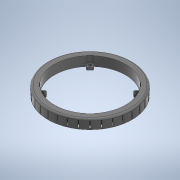
# Autodesk Inventor part: tsop_head_v2
Saved by Autodesk Inventor 2020 (Build 240168000, 168)
## iProperties
Created: 2024-03-11
Part Number: tsop_head_v2
Material: Типовые
Document SubType Name: Modeling
Designer: 4s
Density: 1 g/cm^3
Appearance: Гладкая — черная
Author: 4s
Autodesk Inventor part; units mm, degrees
ref_plane "YZ Plane" through (0, 0, 0) normal (1, 0, 0) x (0, 1, 0)
ref_plane "XZ Plane" through (0, 0, 0) normal (0, 1, 0) x (-1, 0, 0)
ref_plane "XY Plane" through (0, 0, 0) normal (0, 0, 1) x (1, 0, 0)
sketch "Эскиз1" plane through (0, 0, 0) normal (0, 1, 0) x (-1, 0, 0)
  circle A0 centre (0, 0) radius 44 construction
  line L0 (46.1, 2.85) -> (42.7, 2.85)
  line L1 (42.7, 2.85) -> (42.7, -2.85)
  line L2 (42.7, -2.85) -> (46.1, -2.85)
  line L3 (48.1, -0.85) -> (48.1, 0.85)
  line L4 (0, 0) -> (44, 0) construction
  line L5 (0, 0) -> (0, -44) construction
  circle A1 centre (0, 0) radius 49 construction
  circle A2 centre (0, 0) radius 42 construction
  circle A3 centre (0, 0) radius 39 construction
  arc A4 (48.1, 0.85) -> (46.1, 2.85) centre (46.1, 0.85) ccw
  arc A5 (46.1, -2.85) -> (48.1, -0.85) centre (46.1, -0.85) ccw
  line L6 (0, 0) -> (48.1, -0.4908) construction
  line L7 (0, 0) -> (48.1, 0.4908) construction
  line L8 (48.1, 0.4908) -> (48.9974, 0.5)
  line L9 (48.1, -0.4908) -> (48.9974, -0.5)
  line L10 (48.9974, 0.5) -> (49.2908, 0.1398)
  line L11 (49.2908, 0.1398) -> (48.9974, -0.5)
  arc A6 (48.9974, -0.5) -> (48.9974, 0.5) centre (0, 0) ccw
  point P0 (48.1, 2.85)
  point P1 (48.1, -2.85)
  point P2 (49, 0)
  dimension "d0" = 88
  dimension "d1" = 5.7
  dimension "d2" = 1.3
  dimension "d3" = 5.4
  dimension "d4" = 98
  dimension "d5" = 84
  dimension "d6" = 78
  dimension "d16" = 2
  dimension "d17" = 1
  constraints: 24 end point, 11 point on circle, 7 centre point, 6 point on line, 5 coincident, 4 tangent, 2 collinear, 2 horizontal, 2 parallel, 2 perpendicular, 1 equal radius, 1 symmetric about line, 1 other
  measures "d0" diameter of A0
  measures "d1" distance of point (48.1, -2.85) point (48.1, 2.85)
  measures "d2" distance from line of L4.end L1
  measures "d3" distance of L1.end point (48.1, -2.85)
  measures "d4" diameter of A1
  measures "d5" diameter of A2
  measures "d6" diameter of A3
  measures "d16" radius of A4
  measures "d17" distance of L8.end L9.end
sketch "Эскиз2" plane through (0, 0, 0) normal (0, 1, 0) x (-1, 0, 0)
  circle A0 centre (0, 0) radius 49
  circle A1 centre (0, 0) radius 42
  dimension "d7" = 98
  dimension "d8" = 84
  constraints: 2 centre point, 2 coincident
  measures "d7" diameter of A0
  measures "d8" diameter of A1
extrude "Выдавливание1" add sketch "Эскиз2" along normal blind 10
extrude "Выдавливание2" cut sketch "Эскиз1" along normal blind 10 contours A4 L3 A5 L2 L1 L0 | L10 L11 A6
pattern_circular "Круговой массив1" count 32 over 360 about axis through (0, 0, 0) along (0, 1, 0) of "Выдавливание2"
sketch "Эскиз3" plane through (0, 10, 0) normal (0, 1, 0) x (1, 0, 0)
  line L0 (-48.1, -0.85) -> (-48.1, 0.85) construction
  arc A0 (-46.1, 2.85) -> (-48.1, 0.85) centre (-46.1, 0.85) ccw construction
  line L1 (-46.1, 2.85) -> (-42.7, 2.85) construction
  line L2 (-42.7, 2.85) -> (-42.7, -2.85) construction
  line L3 (-42.7, -2.85) -> (-46.1, -2.85) construction
  arc A1 (-48.1, -0.85) -> (-46.1, -2.85) centre (-46.1, -0.85) ccw construction
  line L4 (-47.0099, -10.2175) -> (-47.3416, -8.5502) construction
  arc A2 (-45.7702, -6.1984) -> (-47.3416, -8.5502) centre (-45.38, -8.16) ccw construction
  line L5 (-45.7702, -6.1984) -> (-42.4355, -5.5351) construction
  line L6 (-42.4355, -5.5351) -> (-41.3235, -11.1256) construction
  line L7 (-41.3235, -11.1256) -> (-44.6582, -11.7889) construction
  arc A3 (-47.0099, -10.2175) -> (-44.6582, -11.7889) centre (-45.0484, -9.8273) ccw construction
  line L8 (-44.1133, -19.1924) -> (-44.7639, -17.6218) construction
  arc A4 (-43.6815, -15.0086) -> (-44.7639, -17.6218) centre (-42.9161, -16.8564) ccw construction
  line L9 (-43.6815, -15.0086) -> (-40.5403, -13.7075) construction
  line L10 (-40.5403, -13.7075) -> (-38.359, -18.9736) construction
  line L11 (-38.359, -18.9736) -> (-41.5002, -20.2748) construction
  arc A5 (-44.1133, -19.1924) -> (-41.5002, -20.2748) centre (-42.2656, -18.427) ccw construction
  line L12 (-39.5215, -27.4297) -> (-40.4659, -26.0162) construction
  arc A6 (-39.9141, -23.2421) -> (-40.4659, -26.0162) centre (-38.803, -24.905) ccw construction
  line L13 (-39.9141, -23.2421) -> (-37.0871, -21.3532) construction
  line L14 (-37.0871, -21.3532) -> (-33.9204, -26.0925) construction
  line L15 (-33.9204, -26.0925) -> (-36.7474, -27.9815) construction
  arc A7 (-39.5215, -27.4297) -> (-36.7474, -27.9815) centre (-37.8585, -26.3185) ccw construction
  line L16 (-33.4108, -34.6129) -> (-34.6129, -33.4108) construction
  arc A8 (-34.6129, -30.5824) -> (-34.6129, -33.4108) centre (-33.1987, -31.9966) ccw construction
  line L17 (-34.6129, -30.5824) -> (-32.2087, -28.1782) construction
  line L18 (-32.2087, -28.1782) -> (-28.1782, -32.2087) construction
  line L19 (-28.1782, -32.2087) -> (-30.5824, -34.6129) construction
  arc A9 (-33.4108, -34.6129) -> (-30.5824, -34.6129) centre (-31.9966, -33.1987) ccw construction
  line L20 (-26.0162, -40.4659) -> (-27.4297, -39.5215) construction
  arc A10 (-27.9815, -36.7474) -> (-27.4297, -39.5215) centre (-26.3185, -37.8585) ccw construction
  line L21 (-27.9815, -36.7474) -> (-26.0925, -33.9204) construction
  line L22 (-26.0925, -33.9204) -> (-21.3532, -37.0871) construction
  line L23 (-21.3532, -37.0871) -> (-23.2421, -39.9141) construction
  arc A11 (-26.0162, -40.4659) -> (-23.2421, -39.9141) centre (-24.905, -38.803) ccw construction
  line L24 (-17.6218, -44.7639) -> (-19.1924, -44.1133) construction
  arc A12 (-20.2748, -41.5002) -> (-19.1924, -44.1133) centre (-18.427, -42.2656) ccw construction
  line L25 (-20.2748, -41.5002) -> (-18.9736, -38.359) construction
  line L26 (-18.9736, -38.359) -> (-13.7075, -40.5403) construction
  line L27 (-13.7075, -40.5403) -> (-15.0086, -43.6815) construction
  arc A13 (-17.6218, -44.7639) -> (-15.0086, -43.6815) centre (-16.8564, -42.9161) ccw construction
  line L28 (-8.5502, -47.3416) -> (-10.2175, -47.0099) construction
  arc A14 (-11.7889, -44.6582) -> (-10.2175, -47.0099) centre (-9.8273, -45.0484) ccw construction
  line L29 (-11.7889, -44.6582) -> (-11.1256, -41.3235) construction
  line L30 (-11.1256, -41.3235) -> (-5.5351, -42.4355) construction
  line L31 (-5.5351, -42.4355) -> (-6.1984, -45.7702) construction
  arc A15 (-8.5502, -47.3416) -> (-6.1984, -45.7702) centre (-8.16, -45.38) ccw construction
  line L32 (0.85, -48.1) -> (-0.85, -48.1) construction
  arc A16 (-2.85, -46.1) -> (-0.85, -48.1) centre (-0.85, -46.1) ccw construction
  line L33 (-2.85, -46.1) -> (-2.85, -42.7) construction
  line L34 (-2.85, -42.7) -> (2.85, -42.7) construction
  line L35 (2.85, -42.7) -> (2.85, -46.1) construction
  arc A17 (0.85, -48.1) -> (2.85, -46.1) centre (0.85, -46.1) ccw construction
  line L36 (10.2175, -47.0099) -> (8.5502, -47.3416) construction
  arc A18 (6.1984, -45.7702) -> (8.5502, -47.3416) centre (8.16, -45.38) ccw construction
  line L37 (6.1984, -45.7702) -> (5.5351, -42.4355) construction
  line L38 (5.5351, -42.4355) -> (11.1256, -41.3235) construction
  line L39 (11.1256, -41.3235) -> (11.7889, -44.6582) construction
  arc A19 (10.2175, -47.0099) -> (11.7889, -44.6582) centre (9.8273, -45.0484) ccw construction
  line L40 (19.1924, -44.1133) -> (17.6218, -44.7639) construction
  arc A20 (15.0086, -43.6815) -> (17.6218, -44.7639) centre (16.8564, -42.9161) ccw construction
  line L41 (15.0086, -43.6815) -> (13.7075, -40.5403) construction
  line L42 (13.7075, -40.5403) -> (18.9736, -38.359) construction
  line L43 (18.9736, -38.359) -> (20.2748, -41.5002) construction
  arc A21 (19.1924, -44.1133) -> (20.2748, -41.5002) centre (18.427, -42.2656) ccw construction
  line L44 (27.4297, -39.5215) -> (26.0162, -40.4659) construction
  arc A22 (23.2421, -39.9141) -> (26.0162, -40.4659) centre (24.905, -38.803) ccw construction
  line L45 (23.2421, -39.9141) -> (21.3532, -37.0871) construction
  line L46 (21.3532, -37.0871) -> (26.0925, -33.9204) construction
  line L47 (26.0925, -33.9204) -> (27.9815, -36.7474) construction
  arc A23 (27.4297, -39.5215) -> (27.9815, -36.7474) centre (26.3185, -37.8585) ccw construction
  line L48 (34.6129, -33.4108) -> (33.4108, -34.6129) construction
  arc A24 (30.5824, -34.6129) -> (33.4108, -34.6129) centre (31.9966, -33.1987) ccw construction
  line L49 (30.5824, -34.6129) -> (28.1782, -32.2087) construction
  line L50 (28.1782, -32.2087) -> (32.2087, -28.1782) construction
  line L51 (32.2087, -28.1782) -> (34.6129, -30.5824) construction
  arc A25 (34.6129, -33.4108) -> (34.6129, -30.5824) centre (33.1987, -31.9966) ccw construction
  line L52 (40.4659, -26.0162) -> (39.5215, -27.4297) construction
  arc A26 (36.7474, -27.9815) -> (39.5215, -27.4297) centre (37.8585, -26.3185) ccw construction
  line L53 (36.7474, -27.9815) -> (33.9204, -26.0925) construction
  line L54 (33.9204, -26.0925) -> (37.0871, -21.3532) construction
  line L55 (37.0871, -21.3532) -> (39.9141, -23.2421) construction
  arc A27 (40.4659, -26.0162) -> (39.9141, -23.2421) centre (38.803, -24.905) ccw construction
  line L56 (44.7639, -17.6218) -> (44.1133, -19.1924) construction
  arc A28 (41.5002, -20.2748) -> (44.1133, -19.1924) centre (42.2656, -18.427) ccw construction
  line L57 (41.5002, -20.2748) -> (38.359, -18.9736) construction
  line L58 (38.359, -18.9736) -> (40.5403, -13.7075) construction
  line L59 (40.5403, -13.7075) -> (43.6815, -15.0086) construction
  arc A29 (44.7639, -17.6218) -> (43.6815, -15.0086) centre (42.9161, -16.8564) ccw construction
  line L60 (47.3416, -8.5502) -> (47.0099, -10.2175) construction
  arc A30 (44.6582, -11.7889) -> (47.0099, -10.2175) centre (45.0484, -9.8273) ccw construction
  line L61 (44.6582, -11.7889) -> (41.3235, -11.1256) construction
  line L62 (41.3235, -11.1256) -> (42.4355, -5.5351) construction
  line L63 (42.4355, -5.5351) -> (45.7702, -6.1984) construction
  arc A31 (47.3416, -8.5502) -> (45.7702, -6.1984) centre (45.38, -8.16) ccw construction
  line L64 (48.1, 0.85) -> (48.1, -0.85) construction
  arc A32 (46.1, -2.85) -> (48.1, -0.85) centre (46.1, -0.85) ccw construction
  line L65 (46.1, -2.85) -> (42.7, -2.85) construction
  line L66 (42.7, -2.85) -> (42.7, 2.85) construction
  line L67 (42.7, 2.85) -> (46.1, 2.85) construction
  arc A33 (48.1, 0.85) -> (46.1, 2.85) centre (46.1, 0.85) ccw construction
  line L68 (47.0099, 10.2175) -> (47.3416, 8.5502) construction
  arc A34 (45.7702, 6.1984) -> (47.3416, 8.5502) centre (45.38, 8.16) ccw construction
  line L69 (45.7702, 6.1984) -> (42.4355, 5.5351) construction
  line L70 (42.4355, 5.5351) -> (41.3235, 11.1256) construction
  line L71 (41.3235, 11.1256) -> (44.6582, 11.7889) construction
  arc A35 (47.0099, 10.2175) -> (44.6582, 11.7889) centre (45.0484, 9.8273) ccw construction
  line L72 (44.1133, 19.1924) -> (44.7639, 17.6218) construction
  arc A36 (43.6815, 15.0086) -> (44.7639, 17.6218) centre (42.9161, 16.8564) ccw construction
  line L73 (43.6815, 15.0086) -> (40.5403, 13.7075) construction
  line L74 (40.5403, 13.7075) -> (38.359, 18.9736) construction
  line L75 (38.359, 18.9736) -> (41.5002, 20.2748) construction
  arc A37 (44.1133, 19.1924) -> (41.5002, 20.2748) centre (42.2656, 18.427) ccw construction
  line L76 (39.5215, 27.4297) -> (40.4659, 26.0162) construction
  arc A38 (39.9141, 23.2421) -> (40.4659, 26.0162) centre (38.803, 24.905) ccw construction
  line L77 (39.9141, 23.2421) -> (37.0871, 21.3532) construction
  line L78 (37.0871, 21.3532) -> (33.9204, 26.0925) construction
  line L79 (33.9204, 26.0925) -> (36.7474, 27.9815) construction
  arc A39 (39.5215, 27.4297) -> (36.7474, 27.9815) centre (37.8585, 26.3185) ccw construction
  line L80 (33.4108, 34.6129) -> (34.6129, 33.4108) construction
  arc A40 (34.6129, 30.5824) -> (34.6129, 33.4108) centre (33.1987, 31.9966) ccw construction
  line L81 (34.6129, 30.5824) -> (32.2087, 28.1782) construction
  line L82 (32.2087, 28.1782) -> (28.1782, 32.2087) construction
  line L83 (28.1782, 32.2087) -> (30.5824, 34.6129) construction
  arc A41 (33.4108, 34.6129) -> (30.5824, 34.6129) centre (31.9966, 33.1987) ccw construction
  line L84 (26.0162, 40.4659) -> (27.4297, 39.5215) construction
  arc A42 (27.9815, 36.7474) -> (27.4297, 39.5215) centre (26.3185, 37.8585) ccw construction
  line L85 (27.9815, 36.7474) -> (26.0925, 33.9204) construction
  line L86 (26.0925, 33.9204) -> (21.3532, 37.0871) construction
  line L87 (21.3532, 37.0871) -> (23.2421, 39.9141) construction
  arc A43 (26.0162, 40.4659) -> (23.2421, 39.9141) centre (24.905, 38.803) ccw construction
  line L88 (17.6218, 44.7639) -> (19.1924, 44.1133) construction
  arc A44 (20.2748, 41.5002) -> (19.1924, 44.1133) centre (18.427, 42.2656) ccw construction
  line L89 (20.2748, 41.5002) -> (18.9736, 38.359) construction
  line L90 (18.9736, 38.359) -> (13.7075, 40.5403) construction
  line L91 (13.7075, 40.5403) -> (15.0086, 43.6815) construction
  arc A45 (17.6218, 44.7639) -> (15.0086, 43.6815) centre (16.8564, 42.9161) ccw construction
  line L92 (8.5502, 47.3416) -> (10.2175, 47.0099) construction
  arc A46 (11.7889, 44.6582) -> (10.2175, 47.0099) centre (9.8273, 45.0484) ccw construction
  line L93 (11.7889, 44.6582) -> (11.1256, 41.3235) construction
  line L94 (11.1256, 41.3235) -> (5.5351, 42.4355) construction
  line L95 (5.5351, 42.4355) -> (6.1984, 45.7702) construction
  arc A47 (8.5502, 47.3416) -> (6.1984, 45.7702) centre (8.16, 45.38) ccw construction
  line L96 (-0.85, 48.1) -> (0.85, 48.1) construction
  arc A48 (2.85, 46.1) -> (0.85, 48.1) centre (0.85, 46.1) ccw construction
  line L97 (2.85, 46.1) -> (2.85, 42.7) construction
  line L98 (2.85, 42.7) -> (-2.85, 42.7) construction
  line L99 (-2.85, 42.7) -> (-2.85, 46.1) construction
  arc A49 (-0.85, 48.1) -> (-2.85, 46.1) centre (-0.85, 46.1) ccw construction
  line L100 (-10.2175, 47.0099) -> (-8.5502, 47.3416) construction
  arc A50 (-6.1984, 45.7702) -> (-8.5502, 47.3416) centre (-8.16, 45.38) ccw construction
  line L101 (-6.1984, 45.7702) -> (-5.5351, 42.4355) construction
  line L102 (-5.5351, 42.4355) -> (-11.1256, 41.3235) construction
  line L103 (-11.1256, 41.3235) -> (-11.7889, 44.6582) construction
  arc A51 (-10.2175, 47.0099) -> (-11.7889, 44.6582) centre (-9.8273, 45.0484) ccw construction
  line L104 (-19.1924, 44.1133) -> (-17.6218, 44.7639) construction
  arc A52 (-15.0086, 43.6815) -> (-17.6218, 44.7639) centre (-16.8564, 42.9161) ccw construction
  line L105 (-15.0086, 43.6815) -> (-13.7075, 40.5403) construction
  line L106 (-13.7075, 40.5403) -> (-18.9736, 38.359) construction
  line L107 (-18.9736, 38.359) -> (-20.2748, 41.5002) construction
  arc A53 (-19.1924, 44.1133) -> (-20.2748, 41.5002) centre (-18.427, 42.2656) ccw construction
  line L108 (-27.4297, 39.5215) -> (-26.0162, 40.4659) construction
  arc A54 (-23.2421, 39.9141) -> (-26.0162, 40.4659) centre (-24.905, 38.803) ccw construction
  line L109 (-23.2421, 39.9141) -> (-21.3532, 37.0871) construction
  line L110 (-21.3532, 37.0871) -> (-26.0925, 33.9204) construction
  line L111 (-26.0925, 33.9204) -> (-27.9815, 36.7474) construction
  arc A55 (-27.4297, 39.5215) -> (-27.9815, 36.7474) centre (-26.3185, 37.8585) ccw construction
  line L112 (-34.6129, 33.4108) -> (-33.4108, 34.6129) construction
  arc A56 (-30.5824, 34.6129) -> (-33.4108, 34.6129) centre (-31.9966, 33.1987) ccw construction
  line L113 (-30.5824, 34.6129) -> (-28.1782, 32.2087) construction
  line L114 (-28.1782, 32.2087) -> (-32.2087, 28.1782) construction
  line L115 (-32.2087, 28.1782) -> (-34.6129, 30.5824) construction
  arc A57 (-34.6129, 33.4108) -> (-34.6129, 30.5824) centre (-33.1987, 31.9966) ccw construction
  line L116 (-40.4659, 26.0162) -> (-39.5215, 27.4297) construction
  arc A58 (-36.7474, 27.9815) -> (-39.5215, 27.4297) centre (-37.8585, 26.3185) ccw construction
  line L117 (-36.7474, 27.9815) -> (-33.9204, 26.0925) construction
  line L118 (-33.9204, 26.0925) -> (-37.0871, 21.3532) construction
  line L119 (-37.0871, 21.3532) -> (-39.9141, 23.2421) construction
  arc A59 (-40.4659, 26.0162) -> (-39.9141, 23.2421) centre (-38.803, 24.905) ccw construction
  line L120 (-44.7639, 17.6218) -> (-44.1133, 19.1924) construction
  arc A60 (-41.5002, 20.2748) -> (-44.1133, 19.1924) centre (-42.2656, 18.427) ccw construction
  line L121 (-41.5002, 20.2748) -> (-38.359, 18.9736) construction
  line L122 (-38.359, 18.9736) -> (-40.5403, 13.7075) construction
  line L123 (-40.5403, 13.7075) -> (-43.6815, 15.0086) construction
  arc A61 (-44.7639, 17.6218) -> (-43.6815, 15.0086) centre (-42.9161, 16.8564) ccw construction
  line L124 (-47.3416, 8.5502) -> (-47.0099, 10.2175) construction
  arc A62 (-44.6582, 11.7889) -> (-47.0099, 10.2175) centre (-45.0484, 9.8273) ccw construction
  line L125 (-44.6582, 11.7889) -> (-41.3235, 11.1256) construction
  line L126 (-41.3235, 11.1256) -> (-42.4355, 5.5351) construction
  line L127 (-42.4355, 5.5351) -> (-45.7702, 6.1984) construction
  arc A63 (-47.3416, 8.5502) -> (-45.7702, 6.1984) centre (-45.38, 8.16) ccw construction
  circle A64 centre (0, 0) radius 42 projected
  circle A65 centre (0, 0) radius 49
  constraints: 1 centre point, 1 coincident
extrude "Выдавливание3" add sketch "Эскиз3" along normal blind 1
fillet "Сопряжение1" radius 2 1 edges at (-49, 11, 0)
extrude "Выдавливание4" cut sketch "Эскиз1" along normal blind 9 contours L8 A6 L9 L3
pattern_circular "Круговой массив2" count 32 over 360 about axis through (0, 0, 0) along (0, 1, 0) of "Выдавливание4"
fillet "Сопряжение2" radius 0.5 1 edges at (-47.1758, 9, -9.3838)
sketch "Эскиз4" plane through (0, 0, 0) normal (0, -1, 0) x (1, 0, 0)
  circle A0 centre (0, 0) radius 39 construction
  line L0 (0, 0) -> (-27.5772, -27.5772) construction
  line L1 (0, 0) -> (39, 0) construction
  circle A1 centre (-27.5772, -27.5772) radius 1.7
  line L2 (0, 0) -> (0, -39) construction
  circle A2 centre (27.5772, -27.5772) radius 1.7
  circle A3 centre (-27.5772, 27.5772) radius 1.7
  circle A4 centre (27.5772, 27.5772) radius 1.7
  line L3 (-31.9075, -27.3113) -> (-28.8146, -24.2184)
  line L4 (-27.3113, -31.9075) -> (-24.2184, -28.8146)
  circle A5 centre (0, 0) radius 42 construction
  circle A6 centre (0, 0) radius 47 construction
  circle A7 centre (0, 0) radius 42 construction
  line L5 (-26.6933, -24.2184) -> (-24.2184, -26.6933)
  arc A8 (-24.2184, -28.8146) -> (-24.2184, -26.6933) centre (-25.2791, -27.7539) ccw
  arc A9 (-26.6933, -24.2184) -> (-28.8146, -24.2184) centre (-27.7539, -25.2791) ccw
  arc A10 (-31.9075, -27.3113) -> (-27.3113, -31.9075) centre (0, 0) ccw
  point P0 (-39, 0)
  point P1 (0, 39)
  point P2 (-27.7539, -23.1577)
  point P3 (-23.1577, -27.7539)
  dimension "d27" = 78
  dimension "d28" = 135
  dimension "d29" = 3.4
  dimension "d30" = 6.5
  dimension "d31" = 3
  dimension "d32" = 1.5
  dimension "d33" = 42
  constraints: 12 end point, 11 point on circle, 8 centre point, 5 symmetric about line, 4 point on line, 4 tangent, 2 coincident, 1 equal length, 1 equal radius, 1 horizontal, 1 parallel, 1 vertical, 5 other
  measures "d27" diameter of A0
  measures "d28" angle of L0 L1
  measures "d29" diameter of A1
  measures "d30" distance between parallel lines of L3 L4
  measures "d31" distance from line of L0.end L5
  measures "d32" radius of A8
  measures "d33" radius of A10
extrude "Выдавливание5" add sketch "Эскиз4" along normal blind 0 and the other way blind 2.8 contours L3 A9 L5 A8 L4 A10
pattern_circular "Круговой массив3" count 4 over 360 about axis through (0, 0, 0) along (0, 1, 0) of "Выдавливание5"
sketch "Эскиз5" plane through (0, 0, 0) normal (0, -1, 0) x (1, 0, 0)
  circle A0 centre (0, 0) radius 47 construction
  line L0 (-47.08, -9.8653) -> (-47.9584, -10.0493) construction
  arc A1 (-47.9584, -10.0493) -> (-45.4591, -18.2886) centre (0, 0) ccw construction
  line L1 (-45.4591, -18.2886) -> (-44.6264, -17.9536) construction
  line L2 (-44.6264, -17.9536) -> (-44.7639, -17.6218) construction
  arc A2 (-43.6815, -15.0086) -> (-44.7639, -17.6218) centre (-42.9161, -16.8564) ccw construction
  line L3 (-43.6815, -15.0086) -> (-40.5403, -13.7075) construction
  line L4 (-40.5403, -13.7075) -> (-38.359, -18.9736) construction
  line L5 (-38.359, -18.9736) -> (-41.5002, -20.2748) construction
  arc A3 (-44.1133, -19.1924) -> (-41.5002, -20.2748) centre (-42.2656, -18.427) ccw construction
  line L6 (-44.1133, -19.1924) -> (-44.2508, -18.8606) construction
  line L7 (-44.2508, -18.8606) -> (-45.0764, -19.2125) construction
  arc A4 (-45.0764, -19.2125) -> (-41.0177, -26.8058) centre (0, 0) ccw construction
  line L8 (-41.0177, -26.8058) -> (-40.2664, -26.3148) construction
  line L9 (-40.2664, -26.3148) -> (-40.4659, -26.0162) construction
  arc A5 (-39.9141, -23.2421) -> (-40.4659, -26.0162) centre (-38.803, -24.905) ccw construction
  line L10 (-39.9141, -23.2421) -> (-37.0871, -21.3532) construction
  line L11 (-37.0871, -21.3532) -> (-33.9204, -26.0925) construction
  line L12 (-33.9204, -26.0925) -> (-36.7474, -27.9815) construction
  arc A6 (-39.5215, -27.4297) -> (-36.7474, -27.9815) centre (-37.8585, -26.3185) ccw construction
  line L13 (-39.5215, -27.4297) -> (-39.721, -27.131) construction
  line L14 (-39.721, -27.131) -> (-40.4621, -27.6373) construction
  arc A7 (-40.4621, -27.6373) -> (-35, -34.2929) centre (0, 0) ccw construction
  line L15 (-35, -34.2929) -> (-34.3589, -33.6648) construction
  line L16 (-34.3589, -33.6648) -> (-34.6129, -33.4108) construction
  arc A8 (-34.6129, -30.5824) -> (-34.6129, -33.4108) centre (-33.1987, -31.9966) ccw construction
  line L17 (-34.6129, -30.5824) -> (-32.2087, -28.1782) construction
  line L18 (-32.2087, -28.1782) -> (-28.1782, -32.2087) construction
  line L19 (-28.1782, -32.2087) -> (-30.5824, -34.6129) construction
  arc A9 (-33.4108, -34.6129) -> (-30.5824, -34.6129) centre (-31.9966, -33.1987) ccw construction
  line L20 (-33.4108, -34.6129) -> (-33.6648, -34.3589) construction
  line L21 (-33.6648, -34.3589) -> (-34.2929, -35) construction
  arc A10 (-34.2929, -35) -> (-27.6373, -40.4621) centre (0, 0) ccw construction
  line L22 (-27.6373, -40.4621) -> (-27.131, -39.721) construction
  line L23 (-27.131, -39.721) -> (-27.4297, -39.5215) construction
  arc A11 (-27.9815, -36.7474) -> (-27.4297, -39.5215) centre (-26.3185, -37.8585) ccw construction
  line L24 (-27.9815, -36.7474) -> (-26.0925, -33.9204) construction
  line L25 (-26.0925, -33.9204) -> (-21.3532, -37.0871) construction
  line L26 (-21.3532, -37.0871) -> (-23.2421, -39.9141) construction
  arc A12 (-26.0162, -40.4659) -> (-23.2421, -39.9141) centre (-24.905, -38.803) ccw construction
  line L27 (-26.0162, -40.4659) -> (-26.3148, -40.2664) construction
  line L28 (-26.3148, -40.2664) -> (-26.8058, -41.0177) construction
  arc A13 (-26.8058, -41.0177) -> (-19.2125, -45.0764) centre (0, 0) ccw construction
  line L29 (-19.2125, -45.0764) -> (-18.8606, -44.2508) construction
  line L30 (-18.8606, -44.2508) -> (-19.1924, -44.1133) construction
  arc A14 (-20.2748, -41.5002) -> (-19.1924, -44.1133) centre (-18.427, -42.2656) ccw construction
  line L31 (-20.2748, -41.5002) -> (-18.9736, -38.359) construction
  line L32 (-18.9736, -38.359) -> (-13.7075, -40.5403) construction
  line L33 (-13.7075, -40.5403) -> (-15.0086, -43.6815) construction
  arc A15 (-17.6218, -44.7639) -> (-15.0086, -43.6815) centre (-16.8564, -42.9161) ccw construction
  line L34 (-17.6218, -44.7639) -> (-17.9536, -44.6264) construction
  line L35 (-17.9536, -44.6264) -> (-18.2886, -45.4591) construction
  arc A16 (-18.2886, -45.4591) -> (-10.0493, -47.9584) centre (0, 0) ccw construction
  line L36 (-10.0493, -47.9584) -> (-9.8653, -47.08) construction
  line L37 (-9.8653, -47.08) -> (-10.2175, -47.0099) construction
  arc A17 (-11.7889, -44.6582) -> (-10.2175, -47.0099) centre (-9.8273, -45.0484) ccw construction
  line L38 (-11.7889, -44.6582) -> (-11.1256, -41.3235) construction
  line L39 (-11.1256, -41.3235) -> (-5.5351, -42.4355) construction
  line L40 (-5.5351, -42.4355) -> (-6.1984, -45.7702) construction
  arc A18 (-8.5502, -47.3416) -> (-6.1984, -45.7702) centre (-8.16, -45.38) ccw construction
  line L41 (-8.5502, -47.3416) -> (-8.9024, -47.2715) construction
  line L42 (-8.9024, -47.2715) -> (-9.0685, -48.1535) construction
  arc A19 (-9.0685, -48.1535) -> (-0.5, -48.9974) centre (0, 0) ccw construction
  line L43 (-0.5, -48.9974) -> (-0.4908, -48.1) construction
  line L44 (-0.4908, -48.1) -> (-0.85, -48.1) construction
  arc A20 (-2.85, -46.1) -> (-0.85, -48.1) centre (-0.85, -46.1) ccw construction
  line L45 (-2.85, -46.1) -> (-2.85, -42.7) construction
  line L46 (-2.85, -42.7) -> (2.85, -42.7) construction
  line L47 (2.85, -42.7) -> (2.85, -46.1) construction
  arc A21 (0.85, -48.1) -> (2.85, -46.1) centre (0.85, -46.1) ccw construction
  line L48 (0.85, -48.1) -> (0.4908, -48.1) construction
  line L49 (0.4908, -48.1) -> (0.5, -48.9974) construction
  arc A22 (0.5, -48.9974) -> (9.0685, -48.1535) centre (0, 0) ccw construction
  line L50 (9.0685, -48.1535) -> (8.9024, -47.2715) construction
  line L51 (8.9024, -47.2715) -> (8.5502, -47.3416) construction
  arc A23 (6.1984, -45.7702) -> (8.5502, -47.3416) centre (8.16, -45.38) ccw construction
  line L52 (6.1984, -45.7702) -> (5.5351, -42.4355) construction
  line L53 (5.5351, -42.4355) -> (11.1256, -41.3235) construction
  line L54 (11.1256, -41.3235) -> (11.7889, -44.6582) construction
  arc A24 (10.2175, -47.0099) -> (11.7889, -44.6582) centre (9.8273, -45.0484) ccw construction
  line L55 (10.2175, -47.0099) -> (9.8653, -47.08) construction
  line L56 (9.8653, -47.08) -> (10.0493, -47.9584) construction
  arc A25 (10.0493, -47.9584) -> (18.2886, -45.4591) centre (0, 0) ccw construction
  line L57 (18.2886, -45.4591) -> (17.9536, -44.6264) construction
  line L58 (17.9536, -44.6264) -> (17.6218, -44.7639) construction
  arc A26 (15.0086, -43.6815) -> (17.6218, -44.7639) centre (16.8564, -42.9161) ccw construction
  line L59 (15.0086, -43.6815) -> (13.7075, -40.5403) construction
  line L60 (13.7075, -40.5403) -> (18.9736, -38.359) construction
  line L61 (18.9736, -38.359) -> (20.2748, -41.5002) construction
  arc A27 (19.1924, -44.1133) -> (20.2748, -41.5002) centre (18.427, -42.2656) ccw construction
  line L62 (19.1924, -44.1133) -> (18.8606, -44.2508) construction
  line L63 (18.8606, -44.2508) -> (19.2125, -45.0764) construction
  arc A28 (19.2125, -45.0764) -> (26.8058, -41.0177) centre (0, 0) ccw construction
  line L64 (26.8058, -41.0177) -> (26.3148, -40.2664) construction
  line L65 (26.3148, -40.2664) -> (26.0162, -40.4659) construction
  arc A29 (23.2421, -39.9141) -> (26.0162, -40.4659) centre (24.905, -38.803) ccw construction
  line L66 (23.2421, -39.9141) -> (21.3532, -37.0871) construction
  line L67 (21.3532, -37.0871) -> (26.0925, -33.9204) construction
  line L68 (26.0925, -33.9204) -> (27.9815, -36.7474) construction
  arc A30 (27.4297, -39.5215) -> (27.9815, -36.7474) centre (26.3185, -37.8585) ccw construction
  line L69 (27.4297, -39.5215) -> (27.131, -39.721) construction
  line L70 (27.131, -39.721) -> (27.6373, -40.4621) construction
  arc A31 (27.6373, -40.4621) -> (34.2929, -35) centre (0, 0) ccw construction
  line L71 (34.2929, -35) -> (33.6648, -34.3589) construction
  line L72 (33.6648, -34.3589) -> (33.4108, -34.6129) construction
  arc A32 (30.5824, -34.6129) -> (33.4108, -34.6129) centre (31.9966, -33.1987) ccw construction
  line L73 (30.5824, -34.6129) -> (28.1782, -32.2087) construction
  line L74 (28.1782, -32.2087) -> (32.2087, -28.1782) construction
  line L75 (32.2087, -28.1782) -> (34.6129, -30.5824) construction
  arc A33 (34.6129, -33.4108) -> (34.6129, -30.5824) centre (33.1987, -31.9966) ccw construction
  line L76 (34.6129, -33.4108) -> (34.3589, -33.6648) construction
  line L77 (34.3589, -33.6648) -> (35, -34.2929) construction
  arc A34 (35, -34.2929) -> (40.4621, -27.6373) centre (0, 0) ccw construction
  line L78 (40.4621, -27.6373) -> (39.721, -27.131) construction
  line L79 (39.721, -27.131) -> (39.5215, -27.4297) construction
  arc A35 (36.7474, -27.9815) -> (39.5215, -27.4297) centre (37.8585, -26.3185) ccw construction
  line L80 (36.7474, -27.9815) -> (33.9204, -26.0925) construction
  line L81 (33.9204, -26.0925) -> (37.0871, -21.3532) construction
  line L82 (37.0871, -21.3532) -> (39.9141, -23.2421) construction
  arc A36 (40.4659, -26.0162) -> (39.9141, -23.2421) centre (38.803, -24.905) ccw construction
  line L83 (40.4659, -26.0162) -> (40.2664, -26.3148) construction
  line L84 (40.2664, -26.3148) -> (41.0177, -26.8058) construction
  arc A37 (41.0177, -26.8058) -> (45.0764, -19.2125) centre (0, 0) ccw construction
  line L85 (45.0764, -19.2125) -> (44.2508, -18.8606) construction
  line L86 (44.2508, -18.8606) -> (44.1133, -19.1924) construction
  arc A38 (41.5002, -20.2748) -> (44.1133, -19.1924) centre (42.2656, -18.427) ccw construction
  line L87 (41.5002, -20.2748) -> (38.359, -18.9736) construction
  line L88 (38.359, -18.9736) -> (40.5403, -13.7075) construction
  line L89 (40.5403, -13.7075) -> (43.6815, -15.0086) construction
  arc A39 (44.7639, -17.6218) -> (43.6815, -15.0086) centre (42.9161, -16.8564) ccw construction
  line L90 (44.7639, -17.6218) -> (44.6264, -17.9536) construction
  line L91 (44.6264, -17.9536) -> (45.4591, -18.2886) construction
  arc A40 (45.4591, -18.2886) -> (47.9584, -10.0493) centre (0, 0) ccw construction
  line L92 (47.9584, -10.0493) -> (47.08, -9.8653) construction
  line L93 (47.08, -9.8653) -> (47.0099, -10.2175) construction
  arc A41 (44.6582, -11.7889) -> (47.0099, -10.2175) centre (45.0484, -9.8273) ccw construction
  line L94 (44.6582, -11.7889) -> (41.3235, -11.1256) construction
  line L95 (41.3235, -11.1256) -> (42.4355, -5.5351) construction
  line L96 (42.4355, -5.5351) -> (45.7702, -6.1984) construction
  arc A42 (47.3416, -8.5502) -> (45.7702, -6.1984) centre (45.38, -8.16) ccw construction
  line L97 (47.3416, -8.5502) -> (47.2715, -8.9024) construction
  line L98 (47.2715, -8.9024) -> (48.1535, -9.0685) construction
  arc A43 (48.1535, -9.0685) -> (48.9974, -0.5) centre (0, 0) ccw construction
  line L99 (48.9974, -0.5) -> (48.1, -0.4908) construction
  line L100 (48.1, -0.4908) -> (48.1, -0.85) construction
  arc A44 (46.1, -2.85) -> (48.1, -0.85) centre (46.1, -0.85) ccw construction
  line L101 (46.1, -2.85) -> (42.7, -2.85) construction
  line L102 (42.7, -2.85) -> (42.7, 2.85) construction
  line L103 (42.7, 2.85) -> (46.1, 2.85) construction
  arc A45 (48.1, 0.85) -> (46.1, 2.85) centre (46.1, 0.85) ccw construction
  line L104 (48.1, 0.85) -> (48.1, 0.4908) construction
  line L105 (48.1, 0.4908) -> (48.9974, 0.5) construction
  arc A46 (48.9974, 0.5) -> (48.1535, 9.0685) centre (0, 0) ccw construction
  line L106 (48.1535, 9.0685) -> (47.2715, 8.9024) construction
  line L107 (47.2715, 8.9024) -> (47.3416, 8.5502) construction
  arc A47 (45.7702, 6.1984) -> (47.3416, 8.5502) centre (45.38, 8.16) ccw construction
  line L108 (45.7702, 6.1984) -> (42.4355, 5.5351) construction
  line L109 (42.4355, 5.5351) -> (41.3235, 11.1256) construction
  line L110 (41.3235, 11.1256) -> (44.6582, 11.7889) construction
  arc A48 (47.0099, 10.2175) -> (44.6582, 11.7889) centre (45.0484, 9.8273) ccw construction
  line L111 (47.0099, 10.2175) -> (47.08, 9.8653) construction
  line L112 (47.08, 9.8653) -> (47.9584, 10.0493) construction
  arc A49 (47.9584, 10.0493) -> (45.4591, 18.2886) centre (0, 0) ccw construction
  line L113 (45.4591, 18.2886) -> (44.6264, 17.9536) construction
  line L114 (44.6264, 17.9536) -> (44.7639, 17.6218) construction
  arc A50 (43.6815, 15.0086) -> (44.7639, 17.6218) centre (42.9161, 16.8564) ccw construction
  line L115 (43.6815, 15.0086) -> (40.5403, 13.7075) construction
  line L116 (40.5403, 13.7075) -> (38.359, 18.9736) construction
  line L117 (38.359, 18.9736) -> (41.5002, 20.2748) construction
  arc A51 (44.1133, 19.1924) -> (41.5002, 20.2748) centre (42.2656, 18.427) ccw construction
  line L118 (44.1133, 19.1924) -> (44.2508, 18.8606) construction
  line L119 (44.2508, 18.8606) -> (45.0764, 19.2125) construction
  arc A52 (45.0764, 19.2125) -> (41.0177, 26.8058) centre (0, 0) ccw construction
  line L120 (41.0177, 26.8058) -> (40.2664, 26.3148) construction
  line L121 (40.2664, 26.3148) -> (40.4659, 26.0162) construction
  arc A53 (39.9141, 23.2421) -> (40.4659, 26.0162) centre (38.803, 24.905) ccw construction
  line L122 (39.9141, 23.2421) -> (37.0871, 21.3532) construction
  line L123 (37.0871, 21.3532) -> (33.9204, 26.0925) construction
  line L124 (33.9204, 26.0925) -> (36.7474, 27.9815) construction
  arc A54 (39.5215, 27.4297) -> (36.7474, 27.9815) centre (37.8585, 26.3185) ccw construction
  line L125 (39.5215, 27.4297) -> (39.721, 27.131) construction
  line L126 (39.721, 27.131) -> (40.4621, 27.6373) construction
  arc A55 (40.4621, 27.6373) -> (35, 34.2929) centre (0, 0) ccw construction
  line L127 (35, 34.2929) -> (34.3589, 33.6648) construction
  line L128 (34.3589, 33.6648) -> (34.6129, 33.4108) construction
  arc A56 (34.6129, 30.5824) -> (34.6129, 33.4108) centre (33.1987, 31.9966) ccw construction
  line L129 (34.6129, 30.5824) -> (32.2087, 28.1782) construction
  line L130 (32.2087, 28.1782) -> (28.1782, 32.2087) construction
  line L131 (28.1782, 32.2087) -> (30.5824, 34.6129) construction
  arc A57 (33.4108, 34.6129) -> (30.5824, 34.6129) centre (31.9966, 33.1987) ccw construction
  line L132 (33.4108, 34.6129) -> (33.6648, 34.3589) construction
  line L133 (33.6648, 34.3589) -> (34.2929, 35) construction
  arc A58 (34.2929, 35) -> (27.6373, 40.4621) centre (0, 0) ccw construction
  line L134 (27.6373, 40.4621) -> (27.131, 39.721) construction
  line L135 (27.131, 39.721) -> (27.4297, 39.5215) construction
  arc A59 (27.9815, 36.7474) -> (27.4297, 39.5215) centre (26.3185, 37.8585) ccw construction
  line L136 (27.9815, 36.7474) -> (26.0925, 33.9204) construction
  line L137 (26.0925, 33.9204) -> (21.3532, 37.0871) construction
  line L138 (21.3532, 37.0871) -> (23.2421, 39.9141) construction
  arc A60 (26.0162, 40.4659) -> (23.2421, 39.9141) centre (24.905, 38.803) ccw construction
  line L139 (26.0162, 40.4659) -> (26.3148, 40.2664) construction
  line L140 (26.3148, 40.2664) -> (26.8058, 41.0177) construction
  arc A61 (26.8058, 41.0177) -> (19.2125, 45.0764) centre (0, 0) ccw construction
  line L141 (19.2125, 45.0764) -> (18.8606, 44.2508) construction
  line L142 (18.8606, 44.2508) -> (19.1924, 44.1133) construction
  arc A62 (20.2748, 41.5002) -> (19.1924, 44.1133) centre (18.427, 42.2656) ccw construction
  line L143 (20.2748, 41.5002) -> (18.9736, 38.359) construction
  line L144 (18.9736, 38.359) -> (13.7075, 40.5403) construction
  line L145 (13.7075, 40.5403) -> (15.0086, 43.6815) construction
  arc A63 (17.6218, 44.7639) -> (15.0086, 43.6815) centre (16.8564, 42.9161) ccw construction
  line L146 (17.6218, 44.7639) -> (17.9536, 44.6264) construction
  line L147 (17.9536, 44.6264) -> (18.2886, 45.4591) construction
  arc A64 (18.2886, 45.4591) -> (10.0493, 47.9584) centre (0, 0) ccw construction
  line L148 (10.0493, 47.9584) -> (9.8653, 47.08) construction
  line L149 (9.8653, 47.08) -> (10.2175, 47.0099) construction
  arc A65 (11.7889, 44.6582) -> (10.2175, 47.0099) centre (9.8273, 45.0484) ccw construction
  line L150 (11.7889, 44.6582) -> (11.1256, 41.3235) construction
  line L151 (11.1256, 41.3235) -> (5.5351, 42.4355) construction
  line L152 (5.5351, 42.4355) -> (6.1984, 45.7702) construction
  arc A66 (8.5502, 47.3416) -> (6.1984, 45.7702) centre (8.16, 45.38) ccw construction
  line L153 (8.5502, 47.3416) -> (8.9024, 47.2715) construction
  line L154 (8.9024, 47.2715) -> (9.0685, 48.1535) construction
  arc A67 (9.0685, 48.1535) -> (0.5, 48.9974) centre (0, 0) ccw construction
  line L155 (0.5, 48.9974) -> (0.4908, 48.1) construction
  line L156 (0.4908, 48.1) -> (0.85, 48.1) construction
  arc A68 (2.85, 46.1) -> (0.85, 48.1) centre (0.85, 46.1) ccw construction
  line L157 (2.85, 46.1) -> (2.85, 42.7) construction
  line L158 (2.85, 42.7) -> (-2.85, 42.7) construction
  line L159 (-2.85, 42.7) -> (-2.85, 46.1) construction
  arc A69 (-0.85, 48.1) -> (-2.85, 46.1) centre (-0.85, 46.1) ccw construction
  line L160 (-0.85, 48.1) -> (-0.4908, 48.1) construction
  line L161 (-0.4908, 48.1) -> (-0.5, 48.9974) construction
  arc A70 (-0.5, 48.9974) -> (-9.0685, 48.1535) centre (0, 0) ccw construction
  line L162 (-9.0685, 48.1535) -> (-8.9024, 47.2715) construction
  line L163 (-8.9024, 47.2715) -> (-8.5502, 47.3416) construction
  arc A71 (-6.1984, 45.7702) -> (-8.5502, 47.3416) centre (-8.16, 45.38) ccw construction
  line L164 (-6.1984, 45.7702) -> (-5.5351, 42.4355) construction
  line L165 (-5.5351, 42.4355) -> (-11.1256, 41.3235) construction
  line L166 (-11.1256, 41.3235) -> (-11.7889, 44.6582) construction
  arc A72 (-10.2175, 47.0099) -> (-11.7889, 44.6582) centre (-9.8273, 45.0484) ccw construction
  line L167 (-10.2175, 47.0099) -> (-9.8653, 47.08) construction
  line L168 (-9.8653, 47.08) -> (-10.0493, 47.9584) construction
  arc A73 (-10.0493, 47.9584) -> (-18.2886, 45.4591) centre (0, 0) ccw construction
  line L169 (-18.2886, 45.4591) -> (-17.9536, 44.6264) construction
  line L170 (-17.9536, 44.6264) -> (-17.6218, 44.7639) construction
  arc A74 (-15.0086, 43.6815) -> (-17.6218, 44.7639) centre (-16.8564, 42.9161) ccw construction
  line L171 (-15.0086, 43.6815) -> (-13.7075, 40.5403) construction
  line L172 (-13.7075, 40.5403) -> (-18.9736, 38.359) construction
  line L173 (-18.9736, 38.359) -> (-20.2748, 41.5002) construction
  arc A75 (-19.1924, 44.1133) -> (-20.2748, 41.5002) centre (-18.427, 42.2656) ccw construction
  line L174 (-19.1924, 44.1133) -> (-18.8606, 44.2508) construction
  line L175 (-18.8606, 44.2508) -> (-19.2125, 45.0764) construction
  arc A76 (-19.2125, 45.0764) -> (-26.8058, 41.0177) centre (0, 0) ccw construction
  line L176 (-26.8058, 41.0177) -> (-26.3148, 40.2664) construction
  line L177 (-26.3148, 40.2664) -> (-26.0162, 40.4659) construction
  arc A77 (-23.2421, 39.9141) -> (-26.0162, 40.4659) centre (-24.905, 38.803) ccw construction
  line L178 (-23.2421, 39.9141) -> (-21.3532, 37.0871) construction
  line L179 (-21.3532, 37.0871) -> (-26.0925, 33.9204) construction
  line L180 (-26.0925, 33.9204) -> (-27.9815, 36.7474) construction
  arc A78 (-27.4297, 39.5215) -> (-27.9815, 36.7474) centre (-26.3185, 37.8585) ccw construction
  line L181 (-27.4297, 39.5215) -> (-27.131, 39.721) construction
  line L182 (-27.131, 39.721) -> (-27.6373, 40.4621) construction
  arc A79 (-27.6373, 40.4621) -> (-34.2929, 35) centre (0, 0) ccw construction
  line L183 (-34.2929, 35) -> (-33.6648, 34.3589) construction
  line L184 (-33.6648, 34.3589) -> (-33.4108, 34.6129) construction
  arc A80 (-30.5824, 34.6129) -> (-33.4108, 34.6129) centre (-31.9966, 33.1987) ccw construction
  line L185 (-30.5824, 34.6129) -> (-28.1782, 32.2087) construction
  line L186 (-28.1782, 32.2087) -> (-32.2087, 28.1782) construction
  line L187 (-32.2087, 28.1782) -> (-34.6129, 30.5824) construction
  arc A81 (-34.6129, 33.4108) -> (-34.6129, 30.5824) centre (-33.1987, 31.9966) ccw construction
  line L188 (-34.6129, 33.4108) -> (-34.3589, 33.6648) construction
  line L189 (-34.3589, 33.6648) -> (-35, 34.2929) construction
  arc A82 (-35, 34.2929) -> (-40.4621, 27.6373) centre (0, 0) ccw construction
  line L190 (-40.4621, 27.6373) -> (-39.721, 27.131) construction
  line L191 (-39.721, 27.131) -> (-39.5215, 27.4297) construction
  arc A83 (-36.7474, 27.9815) -> (-39.5215, 27.4297) centre (-37.8585, 26.3185) ccw construction
  line L192 (-36.7474, 27.9815) -> (-33.9204, 26.0925) construction
  line L193 (-33.9204, 26.0925) -> (-37.0871, 21.3532) construction
  line L194 (-37.0871, 21.3532) -> (-39.9141, 23.2421) construction
  arc A84 (-40.4659, 26.0162) -> (-39.9141, 23.2421) centre (-38.803, 24.905) ccw construction
  line L195 (-40.4659, 26.0162) -> (-40.2664, 26.3148) construction
  line L196 (-40.2664, 26.3148) -> (-41.0177, 26.8058) construction
  arc A85 (-41.0177, 26.8058) -> (-45.0764, 19.2125) centre (0, 0) ccw construction
  line L197 (-45.0764, 19.2125) -> (-44.2508, 18.8606) construction
  line L198 (-44.2508, 18.8606) -> (-44.1133, 19.1924) construction
  arc A86 (-41.5002, 20.2748) -> (-44.1133, 19.1924) centre (-42.2656, 18.427) ccw construction
  line L199 (-41.5002, 20.2748) -> (-38.359, 18.9736) construction
  line L200 (-38.359, 18.9736) -> (-40.5403, 13.7075) construction
  line L201 (-40.5403, 13.7075) -> (-43.6815, 15.0086) construction
  arc A87 (-44.7639, 17.6218) -> (-43.6815, 15.0086) centre (-42.9161, 16.8564) ccw construction
  line L202 (-44.7639, 17.6218) -> (-44.6264, 17.9536) construction
  line L203 (-44.6264, 17.9536) -> (-45.4591, 18.2886) construction
  arc A88 (-45.4591, 18.2886) -> (-47.9584, 10.0493) centre (0, 0) ccw construction
  line L204 (-47.9584, 10.0493) -> (-47.08, 9.8653) construction
  line L205 (-47.08, 9.8653) -> (-47.0099, 10.2175) construction
  arc A89 (-44.6582, 11.7889) -> (-47.0099, 10.2175) centre (-45.0484, 9.8273) ccw construction
  line L206 (-44.6582, 11.7889) -> (-41.3235, 11.1256) construction
  line L207 (-41.3235, 11.1256) -> (-42.4355, 5.5351) construction
  line L208 (-42.4355, 5.5351) -> (-45.7702, 6.1984) construction
  arc A90 (-47.3416, 8.5502) -> (-45.7702, 6.1984) centre (-45.38, 8.16) ccw construction
  line L209 (-47.3416, 8.5502) -> (-47.2715, 8.9024) construction
  line L210 (-47.2715, 8.9024) -> (-48.1535, 9.0685) construction
  arc A91 (-48.1535, 9.0685) -> (-48.9974, 0.5) centre (0, 0) ccw construction
  line L211 (-48.9974, 0.5) -> (-48.1, 0.4908) construction
  line L212 (-48.1, 0.4908) -> (-48.1, 0.85) construction
  arc A92 (-46.1, 2.85) -> (-48.1, 0.85) centre (-46.1, 0.85) ccw construction
  line L213 (-46.1, 2.85) -> (-42.7, 2.85) construction
  line L214 (-42.7, 2.85) -> (-42.7, -2.85) construction
  line L215 (-42.7, -2.85) -> (-46.1, -2.85) construction
  arc A93 (-48.1, -0.85) -> (-46.1, -2.85) centre (-46.1, -0.85) ccw construction
  line L216 (-48.1, -0.85) -> (-48.1, -0.4908) construction
  line L217 (-48.1, -0.4908) -> (-48.9974, -0.5) construction
  arc A94 (-48.9974, -0.5) -> (-48.1535, -9.0685) centre (0, 0) ccw construction
  line L218 (-48.1535, -9.0685) -> (-47.2715, -8.9024) construction
  line L219 (-47.2715, -8.9024) -> (-47.3416, -8.5502) construction
  arc A95 (-45.7702, -6.1984) -> (-47.3416, -8.5502) centre (-45.38, -8.16) ccw construction
  line L220 (-45.7702, -6.1984) -> (-42.4355, -5.5351) construction
  line L221 (-42.4355, -5.5351) -> (-41.3235, -11.1256) construction
  line L222 (-41.3235, -11.1256) -> (-44.6582, -11.7889) construction
  arc A96 (-47.0099, -10.2175) -> (-44.6582, -11.7889) centre (-45.0484, -9.8273) ccw construction
  line L223 (-47.0099, -10.2175) -> (-47.08, -9.8653) construction
  arc A97 (-27.3113, -31.9075) -> (27.3113, -31.9075) centre (0, 0) ccw projected
  arc A98 (-31.9075, -27.3113) -> (-27.3113, -31.9075) centre (0, 0) ccw construction
  arc A99 (-31.9075, 27.3113) -> (-31.9075, -27.3113) centre (0, 0) ccw projected
  arc A100 (-27.3113, 31.9075) -> (-31.9075, 27.3113) centre (0, 0) ccw construction
  arc A101 (27.3113, 31.9075) -> (-27.3113, 31.9075) centre (0, 0) ccw projected
  arc A102 (31.9075, 27.3113) -> (27.3113, 31.9075) centre (0, 0) ccw construction
  arc A103 (31.9075, -27.3113) -> (31.9075, 27.3113) centre (0, 0) ccw projected
  arc A104 (27.3113, -31.9075) -> (31.9075, -27.3113) centre (0, 0) ccw construction
  line L224 (27.3113, 31.9075) -> (24.2184, 28.8146) projected
  arc A105 (24.2184, 28.8146) -> (24.2184, 26.6933) centre (25.2791, 27.7539) ccw projected
  line L225 (24.2184, 26.6933) -> (26.6933, 24.2184) projected
  arc A106 (26.6933, 24.2184) -> (28.8146, 24.2184) centre (27.7539, 25.2791) ccw projected
  line L226 (28.8146, 24.2184) -> (31.9075, 27.3113) projected
  arc A107 (31.9075, 27.3113) -> (27.3113, 31.9075) centre (0, 0) ccw construction
  circle A108 centre (27.5772, 27.5772) radius 1.7 projected
  line L227 (31.9075, -27.3113) -> (28.8146, -24.2184) projected
  arc A109 (28.8146, -24.2184) -> (26.6933, -24.2184) centre (27.7539, -25.2791) ccw projected
  line L228 (26.6933, -24.2184) -> (24.2184, -26.6933) projected
  arc A110 (24.2184, -26.6933) -> (24.2184, -28.8146) centre (25.2791, -27.7539) ccw projected
  line L229 (24.2184, -28.8146) -> (27.3113, -31.9075) projected
  arc A111 (27.3113, -31.9075) -> (31.9075, -27.3113) centre (0, 0) ccw construction
  circle A112 centre (27.5772, -27.5772) radius 1.7 projected
  line L230 (-27.3113, -31.9075) -> (-24.2184, -28.8146) projected
  arc A113 (-24.2184, -28.8146) -> (-24.2184, -26.6933) centre (-25.2791, -27.7539) ccw projected
  line L231 (-24.2184, -26.6933) -> (-26.6933, -24.2184) projected
  arc A114 (-26.6933, -24.2184) -> (-28.8146, -24.2184) centre (-27.7539, -25.2791) ccw projected
  line L232 (-28.8146, -24.2184) -> (-31.9075, -27.3113) projected
  arc A115 (-31.9075, -27.3113) -> (-27.3113, -31.9075) centre (0, 0) ccw construction
  circle A116 centre (-27.5772, -27.5772) radius 1.7 projected
  line L233 (-31.9075, 27.3113) -> (-28.8146, 24.2184) projected
  arc A117 (-28.8146, 24.2184) -> (-26.6933, 24.2184) centre (-27.7539, 25.2791) ccw projected
  line L234 (-26.6933, 24.2184) -> (-24.2184, 26.6933) projected
  arc A118 (-24.2184, 26.6933) -> (-24.2184, 28.8146) centre (-25.2791, 27.7539) ccw projected
  line L235 (-24.2184, 28.8146) -> (-27.3113, 31.9075) projected
  arc A119 (-27.3113, 31.9075) -> (-31.9075, 27.3113) centre (0, 0) ccw construction
  circle A120 centre (-27.5772, 27.5772) radius 1.7 projected
  arc A121 (-26.8858, 31.482) -> (-31.482, 26.8858) centre (0, 0) ccw construction
  arc A122 (26.8858, 31.482) -> (-26.8858, 31.482) centre (0, 0) ccw
  arc A123 (31.482, -26.8858) -> (31.482, 26.8858) centre (0, 0) ccw
  arc A124 (31.482, 26.8858) -> (26.8858, 31.482) centre (0, 0) ccw construction
  arc A125 (26.8858, -31.482) -> (31.482, -26.8858) centre (0, 0) ccw construction
  arc A126 (-26.8858, -31.482) -> (26.8858, -31.482) centre (0, 0) ccw
  arc A127 (-31.482, -26.8858) -> (-26.8858, -31.482) centre (0, 0) ccw
  arc A128 (-31.482, 26.8858) -> (-31.482, -26.8858) centre (0, 0) ccw
  point P0 (-27.3113, -31.9075)
  point P1 (-31.9075, 27.3113)
  point P2 (27.3113, 31.9075)
  dimension "d41" = 0.6
  constraints: 16 point on circle, 8 centre point, 8 point on line, 1 coincident
  measures "d41" radial gap between concentric circles of A101 A121
extrude "Выдавливание6" add sketch "Эскиз5" against normal up to surface (11 mm away) contours L230 A126 L229 A97 | L232 A99 L233 A128 | A123 L226 A103 L227 | L235 A101 L224 A122
fillet "Сопряжение3" radius 1 8 edges at (-27.3113, 6.9, -31.9075) (-31.9075, 6.9, -27.3113) (-31.9075, 6.9, 27.3113) (-27.3113, 6.9, 31.9075) (31.9075, 6.9, 27.3113) (27.3113, 6.9, 31.9075) (27.3113, 6.9, -31.9075) (31.9075, 6.9, -27.3113)
sketch "Эскиз6" plane through (-27.131, 0, 39.721) normal (0.8257572, 0, 0.5640257) x (0.5640257, 0, -0.8257572)
  point P0 (48.1025, 0)
extrude "Выдавливание7" add sketch "Эскиз1" along normal blind 1 contours L8 A6 L9 L3
pattern_circular "Круговой массив4" count 32 over 360 about axis through (0, 0, 0) along (0, 1, 0) of "Выдавливание7"
